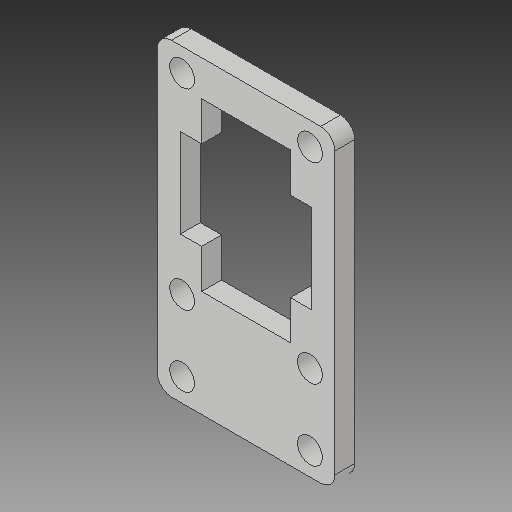
# Autodesk Inventor part: Part17
Saved by Autodesk Inventor 2019.2 (Build 232265000, 265)
## iProperties
Created: 2019-04-01
Part Number: Part17
Material: Generic
Document SubType Name: Modeling
Designer: richard.girt
Mass: 1.84125 g
Surface Area: 21.0909 cm^2
Volume: 1.84125 cm^3
Density: 1 g/cm^3
Appearance: Default
Author: richard.girt
Autodesk Inventor part; units mm, degrees
ref_plane "YZ Plane" through (0, 0, 0) normal (1, 0, 0) x (0, 1, 0)
ref_plane "XZ Plane" through (0, 0, 0) normal (0, 1, 0) x (-1, 0, 0)
ref_plane "XY Plane" through (0, 0, 0) normal (0, 0, 1) x (1, 0, 0)
sketch "Sketch1" plane through (0, 0, 0) normal (0, 0, 1) x (1, 0, 0)
  line L0 (6.25, -11.75) -> (-6.25, -11.75)
  line L1 (-6.25, -11.75) -> (-6.25, 11.75)
  line L2 (-6.25, 11.75) -> (6.25, 11.75)
  line L3 (6.25, 11.75) -> (6.25, -11.75)
  line L4 (6.25, -11.75) -> (-6.25, 11.75) construction
  line L5 (-6.25, -11.75) -> (6.25, 11.75) construction
  line L6 (9.25, 6.25) -> (-9.25, 6.25)
  line L7 (-9.25, 6.25) -> (-9.25, -6.25)
  line L8 (-9.25, -6.25) -> (9.25, -6.25)
  line L9 (9.25, -6.25) -> (9.25, 6.25)
  line L10 (9.25, 6.25) -> (-9.25, -6.25) construction
  line L11 (-9.25, 6.25) -> (9.25, -6.25) construction
  line L12 (-10.5, 16.75) -> (10.5, 16.75)
  line L13 (12.5, 14.75) -> (12.5, -24.75)
  line L14 (10.5, -26.75) -> (-10.5, -26.75)
  line L15 (-12.5, -24.75) -> (-12.5, 14.75)
  line L16 (-9, -13.5) -> (9, -13.5) construction
  line L17 (9, -13.5) -> (9, -23.5) construction
  line L18 (9, -23.5) -> (-9, -23.5) construction
  line L19 (-9, -23.5) -> (-9, -13.5) construction
  circle A0 centre (-9, -23.5) radius 1.75
  circle A1 centre (-9, -13.5) radius 1.75
  circle A2 centre (9, -13.5) radius 1.75
  circle A3 centre (9, -23.5) radius 1.75
  line L20 (-9, 13.5) -> (9, 13.5) construction
  circle A4 centre (-9, 13.5) radius 1.75
  circle A5 centre (9, 13.5) radius 1.75
  arc A6 (-10.5, 16.75) -> (-12.5, 14.75) centre (-10.5, 14.75) ccw
  arc A7 (12.5, 14.75) -> (10.5, 16.75) centre (10.5, 14.75) ccw
  arc A8 (10.5, -26.75) -> (12.5, -24.75) centre (10.5, -24.75) ccw
  arc A9 (-12.5, -24.75) -> (-10.5, -26.75) centre (-10.5, -24.75) ccw
  point P0 (0, 0)
  point P1 (-12.5, 16.75)
  point P2 (12.5, 16.75)
  point P3 (-12.5, -26.75)
  point P4 (0, 16.75)
  point P5 (0, 0)
  point P6 (0, -23.5)
  point P7 (0, 0)
  dimension "d0" = 43.5
  dimension "d1" = 25
  dimension "d2" = 23.5
  dimension "d3" = 12.5
  dimension "d4" = 18.5
  dimension "d5" = 12.5
  dimension "d6" = 16.75
  dimension "d7" = 18
  dimension "d8" = 10
  dimension "d9" = 3.5
  dimension "d10" = 3.25
  dimension "d11" = 3.25
  dimension "d12" = 2
  constraints: 42 end point, 10 centre point, 8 equal radius, 8 midpoint, 8 parallel, 8 point on circle, 8 tangent, 6 coincident, 6 point on line, 5 horizontal, 4 perpendicular, 4 vertical alignment
  measures "d0" distance of point (-12.5, -26.75) point (-12.5, 16.75)
  measures "d1" distance of point (-12.5, 16.75) point (12.5, 16.75)
  measures "d2" distance of L0.end L1.end
  measures "d3" distance of L1.end L2.end
  measures "d4" distance of L7.end L8.end
  measures "d5" distance of L8.end L6.start
  measures "d6" distance from line of L12 point (0, 0)
  measures "d7" distance of L17.end L18.end
  measures "d8" distance of L16.end L17.end
  measures "d9" diameter of A3
  measures "d10" distance from line of L17.end L14
  measures "d11" distance between parallel lines of L20 L12
  measures "d12" radius of A6
extrude "Extrusion1" add sketch "Sketch1" against normal blind 2.8
body "Solid1"
